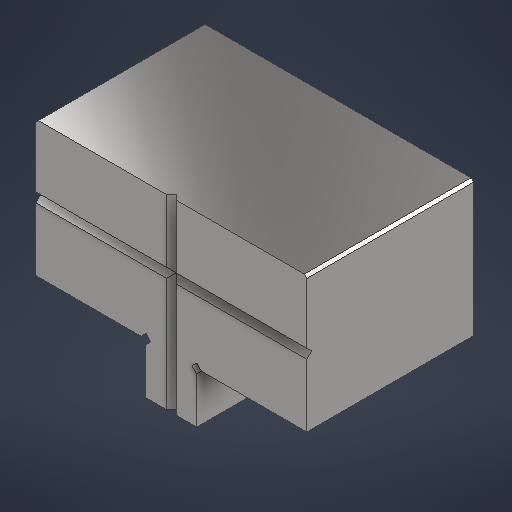
# Autodesk Inventor part: Part4
Saved by Autodesk Inventor 2026 (Build 300175000, 175)
## iProperties
Created: 2026-03-22
Part Number: Part4
Material: Generic
Document SubType Name: Modeling
Designer: Mlinč
Density: 1 g/cm^3
Appearance: Default
Author: Mlinč
Autodesk Inventor part; units mm, degrees
ref_plane "YZ Plane" through (0, 0, 0) normal (1, 0, 0) x (0, 1, 0)
ref_plane "XZ Plane" through (0, 0, 0) normal (0, 1, 0) x (-1, 0, 0)
ref_plane "XY Plane" through (0, 0, 0) normal (0, 0, 1) x (1, 0, 0)
sketch "Sketch1" plane through (0, 0, 0) normal (0, 0, 1) x (1, 0, 0)
  line L0 (0, 0) -> (80, 0)
  line L1 (80, 0) -> (80, 55)
  line L2 (80, 55) -> (0, 55)
  line L3 (0, 55) -> (0, 0)
  dimension "d0" = 55
  dimension "d1" = 80
  constraints: 8 end point, 2 parallel, 1 horizontal, 1 perpendicular
  measures "d0" distance of L2.end L0.start
  measures "d1" distance of L1.end L2.end
extrude "Extrusion1" add sketch "Sketch1" against normal blind 50
sketch "Sketch2" plane through (0, 0, 0) normal (0, 0, 1) x (1, 0, 0)
  line L0 (0, 0) -> (32.5, 0)
  line L1 (32.5, 0) -> (32.5, 15)
  line L2 (32.5, 15) -> (0, 15)
  line L3 (0, 15) -> (0, 0)
  line L4 (80, 55) -> (80, 0) projected
  line L5 (80, 0) -> (47.5, 0)
  line L6 (47.5, 0) -> (47.5, 15)
  line L7 (47.5, 15) -> (80, 15)
  line L8 (80, 15) -> (80, 0)
  dimension "d4" = 15
  dimension "d5" = 15
  constraints: 16 end point, 4 parallel, 2 collinear, 2 horizontal, 2 perpendicular
  measures "d4" distance between parallel lines of L6 L1
  measures "d5" distance of L5.end L6.end
extrude "Extrusion2" cut sketch "Sketch2" against normal through all
sketch "Sketch3" plane through (0, 0, 0) normal (0, 0, 1) x (1, 0, 0)
  line L0 (32.5, 13.5858) -> (31.0858, 15)
  line L1 (31.0858, 15) -> (32.5, 16.4142)
  line L2 (32.5, 16.4142) -> (33.9142, 15)
  line L3 (33.9142, 15) -> (32.5, 13.5858)
  line L4 (32.5, 15) -> (32.5, 0) projected
  line L5 (32.5, 13.5858) -> (32.5, 16.4142) construction
  line L6 (31.0858, 15) -> (33.9142, 15) construction
  line L7 (47.5, 13.5858) -> (48.9142, 15)
  line L8 (48.9142, 15) -> (47.5, 16.4142)
  line L9 (47.5, 16.4142) -> (46.0858, 15)
  line L10 (46.0858, 15) -> (47.5, 13.5858)
  line L11 (47.5, 15) -> (80, 15) projected
  line L12 (47.5, 13.5858) -> (47.5, 16.4142) construction
  line L13 (48.9142, 15) -> (46.0858, 15) construction
  point P0 (0, 0)
  dimension "d8" = 2
  constraints: 24 end point, 5 perpendicular, 4 midpoint, 4 parallel, 2 horizontal
  measures "d8" distance of L1.end L2.end
extrude "Extrusion3" cut sketch "Sketch3" against normal through all
sketch "Sketch4" plane through (80, 55, 0) normal (1, 0, 0) x (0, 0, -1)
  line L0 (-1.4142, -20) -> (0, -18.5858)
  line L1 (0, -18.5858) -> (1.4142, -20)
  line L2 (1.4142, -20) -> (0, -21.4142)
  line L3 (0, -21.4142) -> (-1.4142, -20)
  line L4 (0, -40) -> (0, 0) projected
  line L5 (-1.4142, -20) -> (1.4142, -20) construction
  line L6 (0, -18.5858) -> (0, -21.4142) construction
  line L7 (0, 0) -> (50, 0) projected
  point P0 (0, -55)
  point P1 (0, -20)
  dimension "d11" = 2
  dimension "d12" = 20
  constraints: 12 end point, 3 midpoint, 2 parallel, 2 perpendicular, 1 horizontal
  measures "d11" distance of L0.start L0.end
  measures "d12" distance from line of L7 point (0, -20)
extrude "Extrusion4" cut sketch "Sketch4" against normal through all
sketch "Sketch5" plane through (0, 55, 0) normal (0, 1, 0) x (1, 0, 0)
  line L0 (40, -1.4142) -> (38.5858, 0)
  line L1 (38.5858, 0) -> (40, 1.4142)
  line L2 (40, 1.4142) -> (41.4142, 0)
  line L3 (41.4142, 0) -> (40, -1.4142)
  line L4 (32.5, 0) -> (47.5, 0) projected
  line L5 (40, -1.4142) -> (40, 1.4142) construction
  line L6 (38.5858, 0) -> (41.4142, 0) construction
  point P0 (0, 0)
  point P1 (40, 0)
  dimension "d15" = 2
  constraints: 12 end point, 3 midpoint, 2 parallel, 2 perpendicular, 1 horizontal
  measures "d15" distance of L0.end L1.end
extrude "Extrusion5" cut sketch "Sketch5" against normal through all
sketch "Sketch6" plane through (0, 0, -50) normal (0, 0, -1) x (-1, 0, 0)
  line L0 (-55, 35) -> (-25, 35) construction
  line L1 (-41.4142, 36.4142) -> (-80, 36.4142) projected
  line L2 (-55, 27.5) -> (-25, 27.5)
  line L3 (-25, 42.5) -> (-55, 42.5)
  arc A0 (-55, 42.5) -> (-55, 27.5) centre (-55, 35) ccw
  arc A1 (-25, 27.5) -> (-25, 42.5) centre (-25, 35) ccw
  line L4 (0, 55) -> (-80, 55) projected
  line L5 (-80, 55) -> (-80, 15) projected
  point P0 (0, 0)
  point P1 (-40, 35)
  dimension "d18" = 7.5
  dimension "d19" = 20
  dimension "d20" = 40
  dimension "d21" = 30
  constraints: 8 end point, 4 point on circle, 4 tangent, 2 centre point, 2 parallel, 1 midpoint
  measures "d18" radius of A0
  measures "d19" distance from line of L4 point (-40, 35)
  measures "d20" distance from line of L5 point (-40, 35)
  measures "d21" distance of L3.start L3.end
extrude "Extrusion6" cut sketch "Sketch6" against normal blind 10
sketch "Sketch7" plane through (0, 0, -40) normal (0, 0, -1) x (-1, 0, 0)
  line L0 (-80, 35) -> (-40, 35) projected
  circle A0 centre (-40, 35) radius 7.5
  point P0 (0, 0)
  dimension "d24" = 15
  constraints: 1 centre point
  measures "d24" diameter of A0
extrude "Extrusion7" cut sketch "Sketch7" against normal blind 5
sketch "Sketch8" plane through (0, 0, -40) normal (0, 0, -1) x (-1, 0, 0)
  line L0 (-80, 35) -> (-40, 35) projected
  circle A0 centre (-55, 35) radius 2.5
  line L1 (-40, 35) -> (0, 35) projected
  circle A1 centre (-25, 35) radius 2.5
  point P0 (0, 0)
  dimension "d27" = 5
  dimension "d28" = 15
  dimension "d29" = 15
  constraints: 2 centre point, 2 point on line, 1 equal radius
  measures "d27" diameter of A0
  measures "d28" distance of L0.end A0.centre
  measures "d29" distance of L0.end A1.centre
extrude "Extrusion8" cut sketch "Sketch8" against normal blind 18
thread "Thread1" size "M6x1" class "6H" standard "ANSI Metric M Profile" length 15
thread "Thread2" size "M5x0.8" class "6H" standard "ANSI Metric M Profile" length 15
chamfer "Chamfer1" distance 0.75 angle 45 5 edges at (40, 55, -50) (80, 55, -25) (0, 55, -25) (0, 35, -50) (80, 35, -50)
sketch "Sketch9" plane through (32.5, 0, -50) normal (0, -1, 0) x (1, 0, 0)
  circle A0 centre (7.5, 35) radius 2.5
  circle A1 centre (7.5, 15) radius 2.5
  line L0 (15, 0) -> (0, 0) projected
  point P0 (-32.5, 50)
  point P1 (7.5, 48.5858)
  dimension "d39" = 5
  dimension "d40" = 20
  dimension "d41" = 15
  constraints: 2 centre point, 2 vertical alignment, 1 equal radius
  measures "d39" diameter of A1
  measures "d40" distance of A0.centre A1.centre
  measures "d41" distance from line of L0 A1.centre
extrude "Extrusion9" cut sketch "Sketch9" against normal blind 18
thread "Thread3" size "M6x1" class "6H" standard "ANSI Metric M Profile" length 15
thread "Thread4" size "M6x1" class "6H" standard "ANSI Metric M Profile" length 15
body "Solid1"
